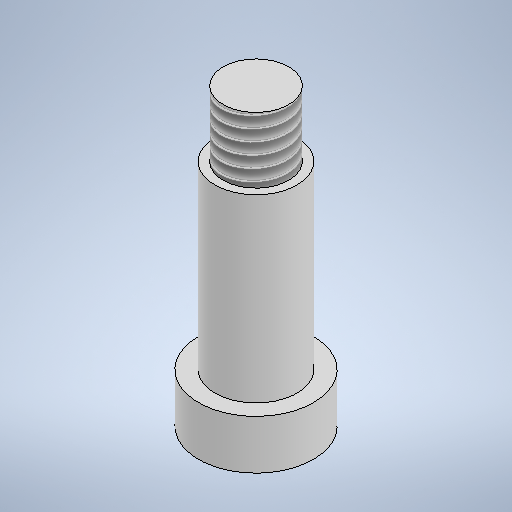
# Autodesk Inventor part: 2053
Saved by Autodesk Inventor 2025 (Build 290162010, 162A)
## iProperties
Created: 2024-06-01
Part Number: 2053
Material: Generic
Document SubType Name: Modeling
Designer: Fabri
Density: 1 g/cm^3
Appearance: Default
Author: Fabri
Autodesk Inventor part; units mm, degrees
ref_plane "YZ Plane" through (0, 0, 0) normal (1, 0, 0) x (0, 1, 0)
ref_plane "XZ Plane" through (0, 0, 0) normal (0, 1, 0) x (-1, 0, 0)
ref_plane "XY Plane" through (0, 0, 0) normal (0, 0, 1) x (1, 0, 0)
sketch "Sketch1" plane through (0, 0, 0) normal (0, 1, 0) x (-1, 0, 0)
  line L0 (0, 0) -> (2, 0)
  line L1 (2, 0) -> (2, -4)
  line L2 (2, -4) -> (2.5, -4)
  line L3 (2.5, -4) -> (2.5, -15)
  line L4 (2.5, -15) -> (3.5, -15)
  line L5 (3.5, -15) -> (3.5, -18)
  line L6 (3.5, -18) -> (0, -18)
  line L7 (0, -18) -> (0, 0)
  dimension "d0" = 3
  dimension "d1" = 11
  dimension "d2" = 4
  dimension "d3" = 7
  dimension "d4" = 5
  dimension "d5" = 4
  constraints: 16 end point, 4 parallel, 3 perpendicular, 1 horizontal
  measures "d0" distance of L4.end L5.end
  measures "d1" distance of L2.end L3.end
  measures "d2" distance of L0.end L1.end
  measures "d3" diameter of L5 L7
  measures "d4" diameter of L3 L7
  measures "d5" diameter of L1 L7
revolve "Revolution1" add sketch "Sketch1" angle 360 about axis through (0, 0, -18) along (0, 0, 1)
thread "Thread1" size "M4x0.7" class "6g" standard "ISO Metric profile" length 12
body "Solid1"
